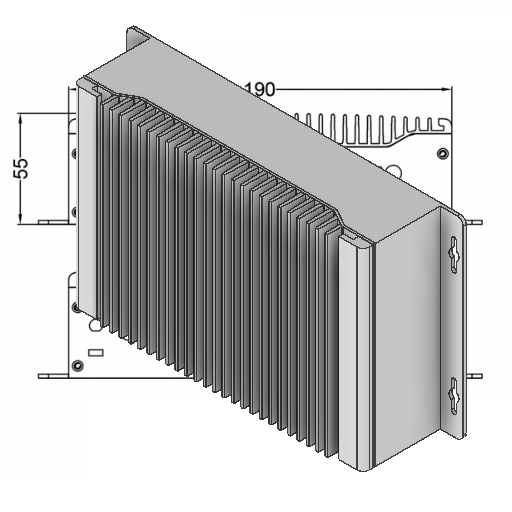
# Autodesk Inventor part: H6-10810
Saved by Autodesk Inventor 2025.2 (Build 292293000, 293)
## iProperties
Created: 2026-04-22
Part Number: H6-10810
Material: Generic
Document SubType Name: Modeling
Designer: valer
Density: 1 g/cm^3
Appearance: Default
Author: valer
Autodesk Inventor part; units mm, degrees
ref_plane "YZ Plane" through (0, 0, 0) normal (1, 0, 0) x (0, 1, 0)
sketch "Base" plane through (0, 0, 0) normal (0, 0, 1) x (1, 0, 0)
  line L0 (-110, -63.15) -> (110, -63.15)
  line L1 (110, -63.15) -> (110, 63.15)
  line L2 (110, 63.15) -> (-110, 63.15)
  line L3 (-110, 63.15) -> (-110, -63.15)
  line L4 (-110, -63.15) -> (110, 63.15) construction
  line L5 (110, -63.15) -> (-110, 63.15) construction
  line L6 (104, -63.15) -> (-104, -63.15)
  line L7 (-104, -63.15) -> (-104, 63.15) construction
  line L8 (-104, 63.15) -> (104, 63.15)
  line L9 (104, 63.15) -> (104, -63.15) construction
  line L10 (104, -63.15) -> (-104, 63.15) construction
  line L11 (-104, -63.15) -> (104, 63.15) construction
  circle A0 centre (-104, 40) radius 3.35
  line L12 (-155.1598, 0) -> (155.1598, 0) construction
  circle A1 centre (-104, -40) radius 3.35
  circle A2 centre (-104, -31.5) radius 1.75
  line L13 (0, -89.5698) -> (0, 89.5698) construction
  circle A3 centre (104, 40) radius 3.35
  circle A4 centre (104, -40) radius 3.35
  line L14 (-104, -40) -> (104, -40) construction
  line L15 (-104, 40) -> (104, 40) construction
  circle A5 centre (-104, -48.5) radius 1.75
  line L16 (-105.75, -31.5) -> (-105.75, -37.1434)
  line L17 (-102.25, -31.5) -> (-102.25, -37.1434)
  line L18 (-105.75, -48.5) -> (-105.75, -42.8566)
  line L19 (-102.25, -48.5) -> (-102.25, -42.8566)
  circle A6 centre (-104, 40) radius 3.35
  circle A7 centre (-104, 31.5) radius 1.75
  circle A8 centre (-104, 48.5) radius 1.75
  line L20 (-105.75, 31.5) -> (-105.75, 37.1434)
  line L21 (-102.25, 31.5) -> (-102.25, 37.1434)
  line L22 (-105.75, 48.5) -> (-105.75, 42.8566)
  line L23 (-102.25, 48.5) -> (-102.25, 42.8566)
  circle A9 centre (104, 40) radius 3.35
  circle A10 centre (104, -40) radius 3.35
  circle A11 centre (104, -31.5) radius 1.75
  circle A12 centre (104, -48.5) radius 1.75
  line L24 (105.75, -31.5) -> (105.75, -37.1434)
  line L25 (102.25, -31.5) -> (102.25, -37.1434)
  line L26 (105.75, -48.5) -> (105.75, -42.8566)
  line L27 (102.25, -48.5) -> (102.25, -42.8566)
  circle A13 centre (104, 31.5) radius 1.75
  line L28 (105.75, 31.5) -> (105.75, 37.1434)
  line L29 (102.25, 31.5) -> (102.25, 37.1434)
  circle A14 centre (104, 48.5) radius 1.75
  line L30 (102.25, 48.5) -> (102.25, 42.8566)
  line L31 (105.75, 48.5) -> (105.75, 42.8566)
  point P0 (0, 0)
  dimension "d0" = 126.3
  dimension "d1" = 220
  dimension "d2" = 208
  dimension "d3" = 6.7
  dimension "d4" = 80
  dimension "d5" = 3.5
  dimension "d6" = 8.5
  constraints: 60 end point, 38 symmetric about line, 15 centre point, 14 point on circle, 5 parallel, 4 midpoint, 4 perpendicular, 3 point on line, 2 horizontal, 2 tangent, 1 vertical, 13 other
  measures "d0" distance of L0.end L1.end
  measures "d1" distance of L1.end L2.end
  measures "d2" distance between parallel lines of L9 L7
  measures "d3" diameter of A0
  measures "d4" distance of L14.start L15.start
  measures "d5" diameter of A2
  measures "d6" distance from line of L14 A2.centre
extrude "BaseFeature" add sketch "Base" along normal blind 2
fillet "BaseFilletsFeature" radius 4 4 edges at (-110, 63.15, 1) (-110, -63.15, 1) (110, -63.15, 1) (110, 63.15, 1)
sketch "Case" plane through (0, 0, 2) normal (0, 0, 1) x (1, 0, 0)
  arc A0 (110, 59.15) -> (106, 63.15) centre (106, 59.15) ccw projected
  line L0 (106, 63.15) -> (-106, 63.15) projected
  arc A1 (-106, 63.15) -> (-110, 59.15) centre (-106, 59.15) ccw projected
  line L1 (-110, 59.15) -> (-110, -59.15) projected
  arc A2 (-110, -59.15) -> (-106, -63.15) centre (-106, -59.15) ccw projected
  line L2 (-106, -63.15) -> (106, -63.15) projected
  arc A3 (106, -63.15) -> (110, -59.15) centre (106, -59.15) ccw projected
  line L3 (110, -59.15) -> (110, 59.15) projected
  arc A4 (102.25, -48.5) -> (105.75, -48.5) centre (104, -48.5) ccw projected
  line L4 (102.25, -48.5) -> (102.25, -42.8566) projected
  arc A5 (102.25, -37.1434) -> (102.25, -42.8566) centre (104, -40) ccw projected
  line L5 (102.25, -37.1434) -> (102.25, -31.5) projected
  arc A6 (105.75, -31.5) -> (102.25, -31.5) centre (104, -31.5) ccw projected
  line L6 (105.75, -31.5) -> (105.75, -37.1434) projected
  arc A7 (105.75, -42.8566) -> (105.75, -37.1434) centre (104, -40) ccw projected
  line L7 (105.75, -42.8566) -> (105.75, -48.5) projected
  arc A8 (102.25, 31.5) -> (105.75, 31.5) centre (104, 31.5) ccw projected
  line L8 (102.25, 31.5) -> (102.25, 37.1434) projected
  arc A9 (102.25, 42.8566) -> (102.25, 37.1434) centre (104, 40) ccw projected
  line L9 (102.25, 42.8566) -> (102.25, 48.5) projected
  arc A10 (105.75, 48.5) -> (102.25, 48.5) centre (104, 48.5) ccw projected
  line L10 (105.75, 48.5) -> (105.75, 42.8566) projected
  arc A11 (105.75, 37.1434) -> (105.75, 42.8566) centre (104, 40) ccw projected
  line L11 (105.75, 37.1434) -> (105.75, 31.5) projected
  line L12 (-105.75, 42.8566) -> (-105.75, 48.5) projected
  arc A12 (-102.25, 48.5) -> (-105.75, 48.5) centre (-104, 48.5) ccw projected
  line L13 (-102.25, 48.5) -> (-102.25, 42.8566) projected
  arc A13 (-102.25, 37.1434) -> (-102.25, 42.8566) centre (-104, 40) ccw projected
  line L14 (-102.25, 37.1434) -> (-102.25, 31.5) projected
  arc A14 (-105.75, 31.5) -> (-102.25, 31.5) centre (-104, 31.5) ccw projected
  line L15 (-105.75, 31.5) -> (-105.75, 37.1434) projected
  arc A15 (-105.75, 42.8566) -> (-105.75, 37.1434) centre (-104, 40) ccw projected
  line L16 (-102.25, -42.8566) -> (-102.25, -48.5) projected
  arc A16 (-105.75, -48.5) -> (-102.25, -48.5) centre (-104, -48.5) ccw projected
  line L17 (-105.75, -48.5) -> (-105.75, -42.8566) projected
  arc A17 (-105.75, -37.1434) -> (-105.75, -42.8566) centre (-104, -40) ccw projected
  line L18 (-105.75, -37.1434) -> (-105.75, -31.5) projected
  arc A18 (-102.25, -31.5) -> (-105.75, -31.5) centre (-104, -31.5) ccw projected
  line L19 (-102.25, -31.5) -> (-102.25, -37.1434) projected
  arc A19 (-102.25, -42.8566) -> (-102.25, -37.1434) centre (-104, -40) ccw projected
  line L20 (-95, -63.15) -> (95, -63.15)
  line L21 (95, -63.15) -> (95, 63.15)
  line L22 (95, 63.15) -> (-95, 63.15)
  line L23 (-95, 63.15) -> (-95, -63.15)
  line L24 (-95, -63.15) -> (95, 63.15) construction
  line L25 (95, -63.15) -> (-95, 63.15) construction
  point P0 (0, 0)
  point P1 (-95, 63.15)
  point P2 (95, -63.15)
  dimension "d10" = 190
  constraints: 12 end point, 2 midpoint, 2 parallel, 1 horizontal, 1 perpendicular, 1 point on line
  measures "d10" distance between parallel lines of L21 L23
extrude "CaseFeature" add sketch "Case" along normal blind 53 contours L21 L2 L23 L0
sketch "Lip" plane through (-106, -63.15, 0) normal (0, -1, 0) x (1, 0, 0)
  line L0 (11, 2) -> (11, 55) projected
  line L1 (11, 44.4) -> (201, 44.4)
  line L2 (201, 2) -> (201, 55) projected
  line L3 (11, 55) -> (201, 55) projected
  line L4 (106, 0) -> (106, 55) construction
  line L5 (11, 55) -> (106, 0) construction
  line L6 (12.9959, 55) -> (42.3595, 38)
  line L7 (42.3595, 38) -> (106, 38)
  line L8 (199.0041, 55) -> (169.6405, 38)
  line L9 (169.6405, 38) -> (106, 38)
  point P0 (31.305, 44.4)
  point P1 (180.695, 44.4)
  dimension "d13" = 10.6
  dimension "d14" = 17
  dimension "d15" = 1
  constraints: 14 end point, 4 point on line, 3 parallel, 2 symmetric about line, 1 midpoint, 1 perpendicular
  measures "d13" distance between parallel lines of L3 L1
  measures "d14" distance between parallel lines of L3 L7
  measures "d15" distance between parallel lines of L5 L6
extrude "LipFeature" cut sketch "Lip" against normal through all
fillet "InsideFilletsFeature" radius 4 4 edges at (-74.695, 0, 44.4) (-63.6405, 0, 38) (63.6405, 0, 38) (74.695, 0, 44.4)
ref_plane "Front" through (-106, -62.9, 0) normal (0, -1, 0) x (1, 0, 0)
ref_plane "Back" through (-106, 63.4, 0) normal (0, 1, 0) x (1, 0, 0)
sketch "Etch" plane through (-106, -62.9, 0) normal (0, -1, 0) x (1, 0, 0)
  line L0 (30.2306, 44.4) -> (11, 44.4) projected
  arc A0 (32.2347, 43.8617) -> (30.2306, 44.4) centre (30.2306, 40.4) ccw projected
  line L1 (41.4297, 38.5383) -> (32.2347, 43.8617) projected
  arc A1 (41.4297, 38.5383) -> (43.4339, 38) centre (43.4339, 42) ccw projected
  line L2 (168.5661, 38) -> (43.4339, 38) projected
  arc A2 (168.5661, 38) -> (170.5703, 38.5383) centre (168.5661, 42) ccw projected
  line L3 (179.7653, 43.8617) -> (170.5703, 38.5383) projected
  arc A3 (181.7694, 44.4) -> (179.7653, 43.8617) centre (181.7694, 40.4) ccw projected
  line L4 (201, 44.4) -> (181.7694, 44.4) projected
  line L5 (11, 44.9) -> (30.2306, 44.9)
  arc A4 (32.4853, 44.2944) -> (30.2306, 44.9) centre (30.2306, 40.4) ccw
  line L6 (32.4853, 44.2944) -> (41.6802, 38.971)
  arc A5 (41.6802, 38.971) -> (43.4339, 38.5) centre (43.4339, 42) ccw
  line L7 (43.4339, 38.5) -> (168.5661, 38.5)
  arc A6 (168.5661, 38.5) -> (170.3198, 38.971) centre (168.5661, 42) ccw
  line L8 (170.3198, 38.971) -> (179.5147, 44.2944)
  arc A7 (181.7694, 44.9) -> (179.5147, 44.2944) centre (181.7694, 40.4) ccw
  line L9 (181.7694, 44.9) -> (200.9987, 44.9)
  line L10 (11, 44.9) -> (11, 44.4)
  line L11 (201, 44.4) -> (200.9987, 44.9)
  point P0 (106, 0)
  dimension "d21" = 0.5
  constraints: 14 end point, 8 point on circle, 4 centre point, 1 vertical, 8 other
  measures "d21" distance between parallel lines of L0 L5
extrude "EtchFeature" add sketch "Etch" against normal blind 126.3
sketch "Lid" plane through (-106, -63.15, 0) normal (0, -1, 0) x (1, 0, 0)
  line L0 (30.2306, 44.9) -> (11, 44.9) projected
  arc A0 (32.4853, 44.2944) -> (30.2306, 44.9) centre (30.2306, 40.4) ccw projected
  line L1 (41.6802, 38.971) -> (32.4853, 44.2944) projected
  arc A1 (41.6802, 38.971) -> (43.4339, 38.5) centre (43.4339, 42) ccw projected
  line L2 (168.5661, 38.5) -> (43.4339, 38.5) projected
  arc A2 (168.5661, 38.5) -> (170.3198, 38.971) centre (168.5661, 42) ccw projected
  line L3 (179.5147, 44.2944) -> (170.3198, 38.971) projected
  arc A3 (181.7694, 44.9) -> (179.5147, 44.2944) centre (181.7694, 40.4) ccw projected
  line L4 (200.9987, 44.9) -> (181.7694, 44.9) projected
  line L5 (11, 45.9) -> (30.2306, 45.9)
  arc A4 (32.9863, 45.1598) -> (30.2306, 45.9) centre (30.2306, 40.4) ccw
  line L6 (32.9863, 45.1598) -> (42.1813, 39.8364)
  arc A5 (42.1813, 39.8364) -> (43.4339, 39.5) centre (43.4339, 42) ccw
  line L7 (43.4339, 39.5) -> (168.5661, 39.5)
  arc A6 (168.5661, 39.5) -> (169.8187, 39.8364) centre (168.5661, 42) ccw
  line L8 (169.8187, 39.8364) -> (179.0137, 45.1598)
  arc A7 (181.7694, 45.9) -> (179.0137, 45.1598) centre (181.7694, 40.4) ccw
  line L9 (181.7694, 45.9) -> (200.9987, 45.9)
  line L10 (11, 45.9) -> (11, 44.9)
  line L11 (200.9987, 45.9) -> (200.9987, 44.9)
  point P0 (106, 0)
  dimension "d24" = 1
  constraints: 14 end point, 8 point on circle, 4 centre point, 1 parallel, 1 vertical, 8 other
  measures "d24" distance between parallel lines of L0 L5
extrude "LidFeature" add sketch "Lid" against normal up to surface (126.55 mm away)
sketch "FrontPanel" plane through (-106, -63.15, 0) normal (0, -1, 0) x (1, 0, 0)
  line L0 (11, 2) -> (11, 44.4) projected
  line L1 (11, 29) -> (14.2936, 29) construction
  line L2 (61, 29) -> (77, 29)
  line L3 (77, 29) -> (77, 15)
  line L4 (77, 15) -> (61, 15)
  line L5 (61, 15) -> (61, 29)
  line L6 (11, 15) -> (201, 15) construction
  line L7 (201, 2) -> (201, 44.4) projected
  line L8 (201, 2) -> (201, 44.4) projected
  line L9 (0, 0) -> (212, 0) projected
  line L10 (82, 29) -> (98, 29)
  line L11 (98, 29) -> (98, 15)
  line L12 (98, 15) -> (82, 15)
  line L13 (82, 15) -> (82, 29)
  line L14 (11, 22) -> (201, 22) construction
  circle A0 centre (51.5, 22) radius 3
  circle A1 centre (40.5, 22) radius 3
  line L15 (21, 15) -> (28, 15)
  line L16 (28, 15) -> (28, 11)
  line L17 (28, 11) -> (21, 11)
  line L18 (21, 11) -> (21, 15)
  circle A2 centre (24.5, 25.5) radius 3.5
  line L19 (24.5, 25.5) -> (24.5, 15) construction
  line L20 (146.5, 28) -> (160.5, 28)
  line L21 (160.5, 28) -> (160.5, 13)
  line L22 (160.5, 13) -> (146.5, 13)
  line L23 (146.5, 13) -> (146.5, 28)
  line L24 (104, 29) -> (111, 29)
  line L25 (111, 29) -> (111, 15)
  line L26 (111, 15) -> (104, 15) construction
  line L27 (104, 15) -> (104, 29)
  line L28 (104, 15) -> (104, 11)
  line L29 (104, 11) -> (107, 11)
  line L30 (107, 11) -> (111, 15)
  circle A3 centre (187.5, 25.5) radius 3.5
  line L31 (106, -9.18) -> (106, 55.08) construction
  line L32 (201, 15) -> (11, 15) construction
  line L33 (184, 15) -> (184, 11)
  line L34 (184, 11) -> (191, 11)
  line L35 (191, 11) -> (191, 15)
  line L36 (184, 15) -> (191, 15)
  line L37 (117, 29) -> (117, 12.5)
  line L38 (117, 12.5) -> (120.2936, 12.5)
  line L39 (120.2936, 12.5) -> (124, 15)
  line L40 (124, 15) -> (124, 25.2936)
  line L41 (124, 25.2936) -> (121.5, 29)
  line L42 (117, 29) -> (121.5, 29)
  line L43 (128, 22) -> (128, 0) construction
  circle A4 centre (171.5, 24) radius 3.5
  line L44 (128, 29) -> (128, 12.5)
  line L45 (135, 25.2936) -> (132.5, 29)
  line L46 (128, 29) -> (132.5, 29)
  line L47 (128, 12.5) -> (131.2936, 12.5)
  line L48 (131.2936, 12.5) -> (135, 15)
  line L49 (135, 15) -> (135, 25.2936)
  point P0 (106, 0)
  point P1 (153.5, 28)
  point P2 (104, 13)
  dimension "d28" = 14
  dimension "d29" = 29
  dimension "d30" = 16
  dimension "d31" = 50
  dimension "d32" = 5
  dimension "d33" = 7
  dimension "d34" = 6
  dimension "d35" = 9.5
  dimension "d37" = 11
  dimension "d38" = 4
  dimension "d39" = 10
  dimension "d40" = 7
  dimension "d41" = 1
  dimension "d42" = 15
  dimension "d43" = 14
  dimension "d44" = 47.5
  dimension "d45" = 6
  dimension "d46" = 7
  dimension "d47" = 4
  dimension "d48" = 3
  dimension "d49" = 13.5
  dimension "d72" = 7
  dimension "d73" = 6
  dimension "d74" = 16.5
  dimension "d75" = 124
  dimension "d76" = 4
  dimension "d77" = 7
  dimension "d78" = 29.5
  dimension "d79" = 2
  dimension "d82" = 11
  constraints: 90 end point, 18 point on line, 14 perpendicular, 10 parallel, 7 horizontal, 6 symmetric about line, 5 centre point, 4 tangent, 3 collinear, 3 equal length, 3 midpoint, 2 vertical, 1 equal radius, 12 other
  measures "d28" distance between parallel lines of L6 L1
  measures "d29" distance between parallel lines of L9 L1
  measures "d30" distance between parallel lines of L3 L5
  measures "d31" distance between parallel lines of L0 L5
  measures "d32" distance between parallel lines of L13 L3
  measures "d33" distance between parallel lines of L6 L14
  measures "d34" diameter of A0
  measures "d35" distance from line of L5 A0.centre
  measures "d37" distance of A0.centre A1.centre
  measures "d38" distance from line of L17.end L6
  measures "d39" distance from line of L0 L15.start
  measures "d40" distance of L15.start L15.end
  measures "d41" distance between parallel lines of L1 L20
  measures "d42" distance between parallel lines of L20 L22
  measures "d43" distance of L21.end L22.end
  measures "d44" distance from line of L7 point (153.5, 28)
  measures "d45" distance between parallel lines of L27 L11
  measures "d46" distance between parallel lines of L25 L27
  measures "d47" distance from line of L28.end L6
  measures "d48" horizontal distance of point (104, 13) L29.end
  measures "d49" distance from line of L7 A3.centre
  measures "d72" distance between parallel lines of L37 L40
  measures "d73" distance between parallel lines of L25 L37
  measures "d74" distance from line of L1 L37.end
  measures "d75" angle of L42 L41
  measures "d76" distance between parallel lines of L40 L43
  measures "d77" diameter of A4
  measures "d78" distance from line of L7 A4.centre
  measures "d79" distance from line of L14 A4.centre
  measures "d82" distance of L37.start L44.start
extrude "FrontPanelFeature" cut sketch "FrontPanel" against normal blind 7
sketch "TopDetail" plane through (-106, -63.15, 0) normal (0, -1, 0) x (1, 0, 0)
  line L0 (30.2306, 45.9) -> (11, 45.9) projected
  line L1 (11, 45.9) -> (11, 48.4)
  arc A0 (15, 52.4) -> (11, 48.4) centre (15, 48.4) ccw
  line L2 (15, 52.4) -> (27, 52.4)
  line L3 (27, 52.4) -> (27, 49.4)
  line L4 (27, 49.4) -> (20.5, 49.4)
  line L5 (20.5, 49.4) -> (20.6153, 45.9)
  line L6 (106, -10.6457) -> (106, 63.8741) construction
  line L7 (106, 85.5) -> (104.667, 38.5) construction
  line L8 (168.5661, 38.5) -> (43.4339, 38.5) projected
  line L9 (11, 48.4) -> (11, 55) construction
  line L10 (11, 55) -> (106, 55) construction
  line L11 (168.5661, 39.5) -> (43.4339, 39.5) projected
  line L12 (201, 55) -> (106, 55) construction
  line L13 (106, 85.5) -> (107.333, 38.5) construction
  line L14 (99.875, 38.5) -> (99.875, 75.1779) construction
  line L15 (104.667, 38.5) -> (105.135, 55)
  line L16 (105.135, 55) -> (106.865, 55)
  line L17 (106.865, 55) -> (107.333, 38.5)
  line L18 (110.792, 38.5) -> (111.26, 55)
  line L19 (111.26, 55) -> (112.99, 55)
  line L20 (112.99, 55) -> (113.458, 38.5)
  line L21 (98.542, 38.5) -> (99.01, 55)
  line L22 (99.01, 55) -> (100.74, 55)
  line L23 (100.74, 55) -> (101.208, 38.5)
  line L24 (116.917, 38.5) -> (117.385, 55)
  line L25 (117.385, 55) -> (119.115, 55)
  line L26 (119.115, 55) -> (119.583, 38.5)
  line L27 (92.417, 38.5) -> (92.885, 55)
  line L28 (92.885, 55) -> (94.615, 55)
  line L29 (94.615, 55) -> (95.083, 38.5)
  line L30 (123.042, 38.5) -> (123.51, 55)
  line L31 (123.51, 55) -> (125.24, 55)
  line L32 (125.24, 55) -> (125.708, 38.5)
  line L33 (86.292, 38.5) -> (86.76, 55)
  line L34 (86.76, 55) -> (88.49, 55)
  line L35 (88.49, 55) -> (88.958, 38.5)
  line L36 (129.167, 38.5) -> (129.635, 55)
  line L37 (129.635, 55) -> (131.365, 55)
  line L38 (131.365, 55) -> (131.833, 38.5)
  line L39 (80.167, 38.5) -> (80.635, 55)
  line L40 (80.635, 55) -> (82.365, 55)
  line L41 (82.365, 55) -> (82.833, 38.5)
  line L42 (135.292, 38.5) -> (135.76, 55)
  line L43 (135.76, 55) -> (137.49, 55)
  line L44 (137.49, 55) -> (137.958, 38.5)
  line L45 (74.042, 38.5) -> (74.51, 55)
  line L46 (74.51, 55) -> (76.24, 55)
  line L47 (76.24, 55) -> (76.708, 38.5)
  line L48 (141.417, 38.5) -> (141.885, 55)
  line L49 (141.885, 55) -> (143.615, 55)
  line L50 (143.615, 55) -> (144.083, 38.5)
  line L51 (67.917, 38.5) -> (68.385, 55)
  line L52 (68.385, 55) -> (70.115, 55)
  line L53 (70.115, 55) -> (70.583, 38.5)
  line L54 (147.542, 38.5) -> (148.01, 55)
  line L55 (148.01, 55) -> (149.74, 55)
  line L56 (149.74, 55) -> (150.208, 38.5)
  line L57 (61.792, 38.5) -> (62.26, 55)
  line L58 (62.26, 55) -> (63.99, 55)
  line L59 (63.99, 55) -> (64.458, 38.5)
  line L60 (153.667, 38.5) -> (154.135, 55)
  line L61 (154.135, 55) -> (155.865, 55)
  line L62 (155.865, 55) -> (156.333, 38.5)
  line L63 (55.667, 38.5) -> (56.135, 55)
  line L64 (56.135, 55) -> (57.865, 55)
  line L65 (57.865, 55) -> (58.333, 38.5)
  line L66 (159.792, 38.5) -> (160.26, 55)
  line L67 (160.26, 55) -> (161.99, 55)
  line L68 (161.99, 55) -> (162.458, 38.5)
  line L69 (49.542, 38.5) -> (50.01, 55)
  line L70 (50.01, 55) -> (51.74, 55)
  line L71 (51.74, 55) -> (52.208, 38.5)
  line L72 (165.917, 38.5) -> (166.385, 55)
  line L73 (166.385, 55) -> (168.115, 55)
  line L74 (168.115, 55) -> (168.583, 38.5)
  line L75 (43.417, 38.5) -> (43.885, 55)
  line L76 (43.885, 55) -> (45.615, 55)
  line L77 (45.615, 55) -> (46.083, 38.5)
  line L78 (172.042, 38.5) -> (172.51, 55)
  line L79 (172.51, 55) -> (174.24, 55)
  line L80 (174.24, 55) -> (174.708, 38.5)
  line L81 (37.292, 38.5) -> (37.76, 55)
  line L82 (37.76, 55) -> (39.49, 55)
  line L83 (39.49, 55) -> (39.958, 38.5)
  line L84 (178.167, 38.5) -> (178.635, 55)
  line L85 (178.635, 55) -> (180.365, 55)
  line L86 (180.365, 55) -> (180.833, 38.5)
  line L87 (31.167, 38.5) -> (31.635, 55)
  line L88 (31.635, 55) -> (33.365, 55)
  line L89 (33.365, 55) -> (33.833, 38.5)
  line L90 (200.9987, 45.9) -> (181.7694, 45.9) projected
  arc A1 (32.9863, 45.1598) -> (30.2306, 45.9) centre (30.2306, 40.4) ccw projected
  line L91 (42.1813, 39.8364) -> (32.9863, 45.1598) projected
  arc A2 (181.7694, 45.9) -> (179.0137, 45.1598) centre (181.7694, 40.4) ccw projected
  line L92 (179.0137, 45.1598) -> (169.8187, 39.8364) projected
  point P0 (106, 0)
  point P1 (23.75, 49.4)
  point P2 (178.3449, 44.7726)
  point P3 (180.6265, 45.7799)
  point P4 (172.1177, 41.1674)
  point P5 (174.5917, 42.5997)
  point P6 (165.9454, 39.5)
  point P7 (168.5546, 39.5)
  point P8 (159.8204, 39.5)
  point P9 (162.4296, 39.5)
  point P10 (153.6954, 39.5)
  point P11 (156.3046, 39.5)
  point P12 (147.5704, 39.5)
  point P13 (150.1796, 39.5)
  point P14 (141.4454, 39.5)
  point P15 (144.0546, 39.5)
  point P16 (135.3204, 39.5)
  point P17 (137.9296, 39.5)
  point P18 (129.1954, 39.5)
  point P19 (131.8046, 39.5)
  point P20 (123.0704, 39.5)
  point P21 (125.6796, 39.5)
  point P22 (116.9454, 39.5)
  point P23 (119.5546, 39.5)
  point P24 (110.8204, 39.5)
  point P25 (113.4296, 39.5)
  point P26 (104.6954, 39.5)
  point P27 (107.3046, 39.5)
  point P28 (98.5704, 39.5)
  point P29 (101.1796, 39.5)
  point P30 (92.4454, 39.5)
  point P31 (95.0546, 39.5)
  point P32 (86.3204, 39.5)
  point P33 (88.9296, 39.5)
  point P34 (80.1954, 39.5)
  point P35 (82.8046, 39.5)
  point P36 (74.0704, 39.5)
  point P37 (76.6796, 39.5)
  point P38 (67.9454, 39.5)
  point P39 (70.5546, 39.5)
  point P40 (61.8204, 39.5)
  point P41 (64.4296, 39.5)
  point P42 (55.6954, 39.5)
  point P43 (58.3046, 39.5)
  point P44 (49.5704, 39.5)
  point P45 (52.1796, 39.5)
  point P46 (43.4454, 39.5)
  point P47 (46.0546, 39.5)
  point P48 (37.4083, 42.5997)
  point P49 (39.8823, 41.1674)
  point P50 (31.3735, 45.7799)
  point P51 (33.6551, 44.7726)
  dimension "d52" = 6.5
  dimension "d53" = 4
  dimension "d54" = 12
  dimension "d55" = 3.5
  dimension "d56" = 6.5
  dimension "d57" = 47
  dimension "d58" = 15.5
  dimension "d59" = 1.333
  dimension "d60" = 6.125
  dimension "d63" = 6.125
  constraints: 172 end point, 8 point on line, 4 vertical, 3 horizontal, 2 midpoint, 2 point on circle, 2 symmetric about line, 2 tangent, 1 centre point, 1 perpendicular, 169 other
  measures "d52" distance between parallel lines of L0 L2
  measures "d53" radius of A0
  measures "d54" distance of L2.start L2.end
  measures "d55" distance from line of L0 point (23.75, 49.4)
  measures "d56" horizontal distance of L2.end L4.end
  measures "d57" distance from line of L8 L7.start
  measures "d59" distance from line of L6 L7.end
  measures "d60" distance between parallel lines of L6 L14
  measures "d63" distance of L7.end L18.start
extrude "TopDetailSidesFeature" add sketch "TopDetail" against normal up to surface (126.3 mm away) contours L0 L1 A0 L2 L3 L4 L5
mirror "TopDetailSidesMirrorFeature" about plane through (0, 0, 0) normal (1, 0, 0) of "TopDetailSidesFeature"
extrude "HeatsinkFeature" add sketch "TopDetail" against normal up to surface (126.3 mm away) contours L11 L75 L76 L77 | L72 L73 L74 L11 | L11 L66 L67 L68 | L11 L60 L61 L62 | L11 L54 L55 L56 | L11 L48 L49 L50 | L11 L42 L43 L44 | L11 L36 L37 L38 | L11 L30 L31 L32 | L11 L24 L25 L26 | L11 L18 L19 L20 | L11 L15 L16 L17 | L11 L21 L22 L23 | L11 L27 L28 L29 | L11 L33 L34 L35 | L11 L39 L40 L41 | L11 L45 L46 L47 | L11 L51 L52 L53 | L11 L57 L58 L59 | L11 L63 L64 L65 | L11 L69 L70 L71 | L78 L79 L80 L92 | L81 L82 L83 L91 | L84 L85 L86 A2 L92 | L87 L88 L89 L91 A1
equation "\"d50\" = d77"
equation "\"d63\" = d60"
body "Solid1"
